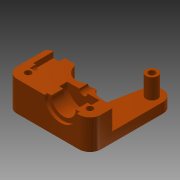
# Autodesk Inventor part: EXTRUDER BODY
Saved by Autodesk Inventor 2013 (Build 170138000, 138)
## iProperties
Created: 2014-06-22
Part Number: EXTRUDER BODY
Material: Generic
Document SubType Name: Modeling
Designer: employee
Density: 1 g/cm^3
d0: 13.500 mm
d2: 31.000 mm
d3: 42.000 mm
d4: 3.100 mm
d5: 15.000 mm
d6: 0.00 deg
d7: 10.795 mm
d9: 8.500 mm
d11: 1.750 mm
d12: 2.000 mm
d13: 10.000 mm
d14: 0.00 deg
d15: 6.273 mm
d16: 12.200 mm
d17: 7.400 mm
d18: 0.00 deg
d19: 16.200 mm
d21: 4.000 mm
d22: 0.00 deg
d24: 16.200 mm
d27: 1.500 mm
d28: 0.00 deg
d29: 4.100 mm
d32: 0.00 deg
d33: 31.000 mm
d34: 6.000 mm
d36: 0.00 deg
d37: 5.700 mm
d38: 15.500 mm
d39: 10.000 mm
d40: 0.00 deg
d41: 3.200 mm
d43: 3.000 mm
d44: 0.00 deg
d45: 5.500 mm
d46: 2.000 mm
d47: 5.800 mm
d50: 10.000 mm
d51: 0.00 deg
d52: 3.200 mm
d55: 0.00 deg
Author: employee
Autodesk Inventor part; units mm, degrees
ref_plane "YZ Plane" through (0, 0, 0) normal (1, 0, 0) x (0, 1, 0)
ref_plane "XZ Plane" through (0, 0, 0) normal (0, 1, 0) x (-1, 0, 0)
ref_plane "XY Plane" through (0, 0, 0) normal (0, 0, 1) x (1, 0, 0)
sketch "Sketch1" plane through (0, 0, 0) normal (0, 0, 1) x (1, 0, 0)
  line L0 (-15.5, 15.5) -> (15.5, 15.5) construction
  line L1 (15.5, 15.5) -> (15.5, -15.5) construction
  line L2 (15.5, -15.5) -> (-15.5, -15.5) construction
  line L3 (-15.5, -15.5) -> (-15.5, 15.5) construction
  circle A0 centre (0, 0) radius 6.75
  line L4 (-21, -21) -> (-21, 21)
  line L5 (-21, 21) -> (21, 21)
  line L6 (21, 21) -> (21, -21)
  line L7 (21, -21) -> (-21, -21)
  circle A1 centre (-15.5, -15.5) radius 1.55
  circle A2 centre (15.5, -15.5) radius 1.55
  dimension "d0" = 13.5
  dimension "d2" = 31
  dimension "d3" = 42
  dimension "d4" = 3.1
  constraints: 16 end point, 5 coincident, 3 centre point, 2 horizontal, 1 equal radius, 18 other
  measures "d0" diameter of A0
  measures "d2" distance of L1.end L2.end
  measures "d3" distance of L6.end L4.start
  measures "d4" diameter of A1
extrude "Extrusion1" add sketch "Sketch1" along normal blind 15
sketch "Sketch2" plane through (0, 0, 15) normal (0, 0, 1) x (1, 0, 0)
  circle A0 centre (0, 0) radius 6.75 projected
  line L0 (-21, 21) -> (-21, -21) projected
  line L1 (21, -21) -> (21, 21) projected
  line L2 (21, 21) -> (-21, 21) projected
  circle A1 centre (0, 0) radius 5.3975
  circle A2 centre (6.2725, 0) radius 0.875
  circle A3 centre (14.7725, 0) radius 7.625
  line L3 (6.2725, 0) -> (6.2725, -2.4936)
  arc A4 (7.1541, -4.0797) -> (5.4631, -3.9644) centre (6.2725, -4.5517) ccw
  arc A5 (7.1541, -4.0797) -> (14.7725, -8.642) centre (14.7725, 0) ccw
  arc A6 (21, 5.9919) -> (6.4006, -2.1436) centre (14.7725, 0) ccw
  line L4 (14.7725, -8.642) -> (21, -8.642)
  line L5 (-6.75, 0) -> (-21, 0)
  dimension "d7" = 10.795
  dimension "d9" = 8.5
  dimension "d11" = 1.75
  dimension "d12" = 2
  constraints: 11 point on circle, 6 centre point, 6 end point, 5 tangent, 2 coincident, 2 horizontal alignment, 2 perpendicular, 2 point on line, 1 horizontal, 1 midpoint, 1 vertical alignment
  measures "d7" diameter of A1
  measures "d9" distance of L3.start A3.centre
  measures "d11" diameter of A2
  measures "d12" diameter of A4
extrude "Extrusion2" cut sketch "Sketch2" against normal blind 10 contours L5 L0 L2 L1 A6 A0 | A0 A2 A3 L1 L4 A5 A4 | A6 L1 A3 A2 A0 | A2 A0 | A3 L1 picked at (15.7085, -1.9503)
sketch "Sketch3" plane through (-21, -21, 0) normal (0, -1, 0) x (1, 0, 0)
  line L0 (0, 15) -> (42, 15) projected
  circle A0 centre (27.2725, 15) radius 6.1
  point P0 (21, 0)
  dimension "d15" = 6.2725
  dimension "d16" = 12.2
  constraints: 1 centre point, 1 point on line
  measures "d15" horizontal distance of A0.centre point (21, 0)
  measures "d16" diameter of A0
extrude "Extrusion3" cut sketch "Sketch3" against normal blind 7.4
sketch "Sketch4" plane through (-21, -13.6, 0) normal (0, -1, 0) x (1, 0, 0)
  arc A0 (21.1725, 15) -> (33.3725, 15) centre (27.2725, 15) ccw projected
  circle A1 centre (27.2725, 15) radius 8.1
  point P0 (21, 0)
  dimension "d19" = 16.2
  constraints: 1 centre point, 1 coincident
  measures "d19" diameter of A1
extrude "Extrusion4" cut sketch "Sketch4" against normal blind 4
sketch "Sketch5" plane through (-21, -21, 0) normal (0, -1, 0) x (1, 0, 0)
  arc A0 (21.1725, 15) -> (33.3725, 15) centre (27.2725, 15) ccw projected
  circle A1 centre (27.2725, 15) radius 8.1
  point P0 (21, 0)
  dimension "d24" = 16.2
  constraints: 1 centre point, 1 coincident
  measures "d24" diameter of A1
extrude "Extrusion5" cut sketch "Sketch5" against normal blind 1.5
sketch "Sketch6" plane through (-21, -9.6, 0) normal (0, -1, 0) x (1, 0, 0)
  arc A0 (19.1725, 15) -> (35.3725, 15) centre (27.2725, 15) ccw projected
  circle A1 centre (27.2725, 15) radius 2.05
  point P0 (21, 0)
  dimension "d29" = 4.1
  constraints: 1 centre point, 1 coincident
  measures "d29" diameter of A1
extrude "Extrusion6" cut sketch "Sketch6" against normal through all
sketch "Sketch7" plane through (0, 0, 5) normal (0, 0, 1) x (1, 0, 0)
  line L0 (-21, 0) -> (-21, 21) projected
  line L1 (-6.75, 0) -> (-21, 0) projected
  arc A0 (5.4631, -3.9644) -> (-6.75, 0) centre (0, 0) ccw projected
  arc A1 (7.1541, -4.0797) -> (5.4631, -3.9644) centre (6.2725, -4.5517) ccw projected
  arc A2 (7.1541, -4.0797) -> (14.7725, -8.642) centre (14.7725, 0) ccw projected
  line L2 (21, -8.642) -> (14.7725, -8.642) projected
  line L3 (21, 21) -> (21, -8.642) projected
  line L4 (-21, 21) -> (21, 21) projected
  line L5 (6.6254, -1.2908) -> (10.1015, 16.5517)
  arc A3 (21, 15.5) -> (10.1015, 16.5517) centre (15.5, 15.5) ccw
  circle A4 centre (15.5, -15.5) radius 1.55 projected
  circle A5 centre (15.5, 15.5) radius 3
  dimension "d33" = 31
  dimension "d34" = 6
  constraints: 3 point on circle, 3 tangent, 2 centre point, 2 end point, 1 coincident, 1 point on line, 1 vertical alignment
  measures "d33" distance of A3.centre A4.centre
  measures "d34" diameter of A5
extrude "Extrusion7" cut sketch "Sketch7" against normal through all contours L0 L4 A3 L5 A0 L1 | L4 L3 A3
sketch "Sketch8" plane through (-21, 0, 15) normal (0, 1, 0) x (1, 0, 0)
  line L0 (14.25, 0) -> (0, 0) projected
  line L1 (2.65, 2.85) -> (8.35, 2.85)
  line L2 (8.35, 2.85) -> (8.35, -2.85)
  line L3 (8.35, -2.85) -> (2.65, -2.85)
  line L4 (2.65, -2.85) -> (2.65, 2.85)
  point P0 (21, 15)
  point P1 (5.5, 0)
  dimension "d37" = 5.7
  dimension "d38" = 15.5
  constraints: 8 end point, 1 horizontal, 1 point on line, 9 other
  measures "d37" distance of L3.end L1.start
  measures "d38" horizontal distance of point (5.5, 0) point (21, 15)
extrude "Extrusion8" cut sketch "Sketch8" against normal blind 10
sketch "Sketch9" plane through (-21, -10, 15) normal (0, 1, 0) x (1, 0, 0)
  line L0 (8.35, 0) -> (2.65, 0) projected
  circle A0 centre (5.5, 0) radius 1.6
  point P0 (21, 15)
  dimension "d41" = 3.2
  constraints: 1 centre point, 1 midpoint
  measures "d41" diameter of A0
extrude "Extrusion9" cut sketch "Sketch9" against normal blind 3
fillet "Fillet1" radius 5.5 2 edges at (-21, -21, 7.5) (21, -21, 7.5)
fillet "Fillet2" radius 2 3 edges at (-21, 0, 7.5) (-6.75, 0, 7.5) (21, -8.642, 10)
sketch "Sketch10" plane through (0, 0, 5) normal (0, 0, 1) x (1, 0, 0)
  arc A0 (21, 15.5) -> (10.1015, 16.5517) centre (15.5, 15.5) ccw projected
  circle A1 centre (15.5, 15.5) radius 2.9
  dimension "d47" = 5.8
  constraints: 1 centre point, 1 coincident
  measures "d47" diameter of A1
extrude "Extrusion10" add sketch "Sketch10" along normal blind 10
sketch "Sketch11" plane through (15.5, 15.5, 15) normal (0, 0, 1) x (1, 0, 0)
  circle A0 centre (0, 0) radius 2.9 projected
  circle A1 centre (0, 0) radius 1.6
  point P0 (-15.5, -15.5)
  dimension "d52" = 3.2
  constraints: 1 centre point, 1 coincident
  measures "d52" diameter of A1
extrude "Extrusion11" cut sketch "Sketch11" against normal through all contours A1
body "Solid1"
